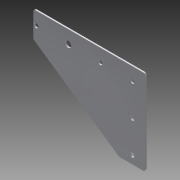
# Autodesk Inventor part: Corner-Tower-Brace Upper
Saved by Autodesk Inventor 2015 SP1 (Build 190203100, 203)
## iProperties
Created: 2015-01-20
Part Number: Corner-Tower-Brace Upper
Material: Aluminum 6061
Document SubType Name: Modeling
Designer: Owner
Density: 2.7 g/cm^3
Appearance: Aluminum - Flat
Mass: 107.392 g
Surface Area: 363.611 cm^2
Volume: 39.7748 cm^3
Author: Owner
Autodesk Inventor part; units mm, degrees
ref_plane "YZ Plane" through (0, 0, 0) normal (1, 0, 0) x (0, 1, 0)
ref_plane "XZ Plane" through (0, 0, 0) normal (0, 1, 0) x (-1, 0, 0)
ref_plane "XY Plane" through (0, 0, 0) normal (0, 0, 1) x (1, 0, 0)
sketch "Sketch1" plane through (0, 0, 0) normal (0, 0, 1) x (1, 0, 0)
  line L0 (0, 0) -> (-41.402, 0)
  line L1 (-41.402, 0) -> (-177.8, 93.599)
  line L2 (-177.8, 93.599) -> (-177.8, 135.001)
  line L3 (-177.8, 135.001) -> (0, 135.001)
  line L4 (0, 135.001) -> (0, 0)
  circle A0 centre (-20.701, 12.7) radius 3.3655
  circle A1 centre (-20.701, 63.5) radius 3.3655
  circle A2 centre (-20.701, 114.3) radius 3.3655
  circle A3 centre (-71.501, 114.3) radius 3.3655
  circle A4 centre (-122.301, 114.3) radius 3.3655
  circle A5 centre (-173.101, 114.3) radius 3.3655
  dimension "d0" = 41.402
  dimension "d1" = 41.402
  dimension "d2" = 177.8
  dimension "d3" = 135.001
  dimension "d4" = 6.731
  dimension "d6" = 20.701
  dimension "d9" = 50.8
  dimension "d14" = 20.701
  dimension "d15" = 20.701
  dimension "d16" = 50.8
  dimension "d17" = 12.7
  dimension "d20" = 50.8
  dimension "d25" = 4.699
  constraints: 10 end point, 6 centre point, 3 perpendicular, 2 horizontal, 1 vertical, 10 other
  measures "d0" distance of L0.start L0.end
  measures "d1" distance of L1.end L2.end
  measures "d2" distance between parallel lines of L2 L4
  measures "d3" distance between parallel lines of L0 L3
  measures "d4" diameter of A0
  measures "d6" distance from line of A0.centre L4
  measures "d9" distance of A0.centre A1.centre
  measures "d14" distance from line of A2.centre L4
  measures "d15" distance from line of L3 A2.centre
  measures "d16" distance of A2.centre A1.centre
  measures "d17" distance from line of A0.centre L0
  measures "d20" distance of A2.centre A3.centre
  measures "d25" distance from line of L2 A5.centre
extrude "Extrusion1" add sketch "Sketch1" along normal blind 2.286
fillet "Fillet1" radius 3.175 5 edges at (0, 135.001, 1.143) (0, 0, 1.143) (-41.402, 0, 1.143) (-177.8, 93.599, 1.143) (-177.8, 135.001, 1.143)
sketch "Sketch2" plane through (0, 0, 2.286) normal (0, 0, 1) x (1, 0, 0)
  circle A0 centre (-122.301, 114.3) radius 3.3655 construction
  circle A1 centre (-122.301, 114.3) radius 4.953
  point P0 (0, 0)
  dimension "d29" = 1.5875
  constraints: 1 centre point, 1 coincident
  measures "d29" radial gap between concentric circles of A0 A1
extrude "Extrusion2" cut sketch "Sketch2" against normal through all
body "Solid1"
